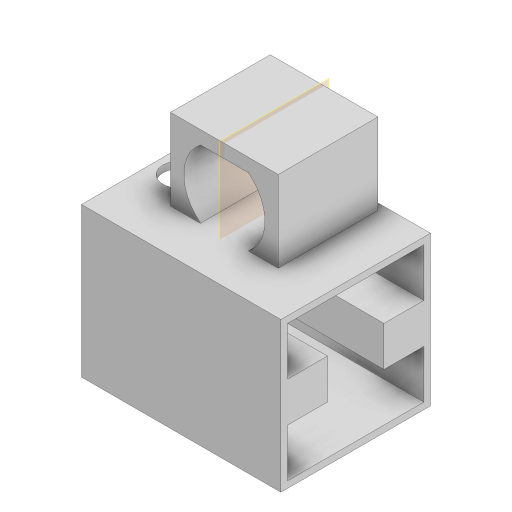
# Autodesk Inventor part: motor mount left
Saved by Autodesk Inventor 2023 (Build 270158000, 158)
## iProperties
Created: 2023-07-19
Part Number: motor mount left
Material: Generic
Document SubType Name: Modeling
Designer: Juyoung Han
Density: 1 g/cm^3
Appearance: Default
Author: Juyoung Han
Autodesk Inventor part; units mm, degrees
ref_plane "YZ Plane" through (0, 0, 0) normal (1, 0, 0) x (0, 1, 0)
ref_plane "XZ Plane" through (0, 0, 0) normal (0, 1, 0) x (-1, 0, 0)
ref_plane "XY Plane" through (0, 0, 0) normal (0, 0, 1) x (1, 0, 0)
sketch "Sketch4" plane through (0, 0, 0) normal (0, 0, 1) x (1, 0, 0)
  arc A0 (2.5, 0) -> (2.5, -10.2) centre (6.452, -5.1) ccw
  arc A1 (9.7, -10.2) -> (9.7, 0) centre (5.748, -5.1) ccw
  line L0 (-2, 2) -> (14.2, 2)
  line L1 (14.2, 2) -> (14.2, -10.2)
  line L2 (-2, -10.2) -> (-2, 2)
  line L3 (-2, -10.2) -> (2.5, -10.2)
  line L4 (9.7, -10.2) -> (14.2, -10.2)
  line L5 (2.5, 0) -> (9.7, 0)
  point P0 (0, 0)
  point P1 (6.1, 0)
  point P2 (6.1, -10.2)
  dimension "d50" = 3.6
  dimension "d51" = 3.6
  dimension "d52" = 3.6
  dimension "d53" = 3.6
  constraints: 12 end point, 4 point on circle, 2 centre point, 1 horizontal, 1 parallel, 1 perpendicular, 1 point on line
  measures "d50" distance of L5.start point (6.1, 0)
  measures "d51" distance of point (6.1, 0) L5.end
  measures "d52" distance of point (6.1, -10.2) L3.end
  measures "d53" distance of point (6.1, -10.2) L4.start
extrude "Extrusion4" add sketch "Sketch4" along normal blind 15
ref_plane "Work Plane2" through (6.1, -10.2, 0) normal (1, 0, 0) x (0, 0, -1)
sketch "Sketch5" plane through (6.1, -10.2, 0) normal (1, 0, 0) x (0, 0, -1)
  line L0 (0, 0) -> (0, 12.2) projected
  line L1 (0, 12.2) -> (-15, 12.2) projected
  line L2 (-15, 0) -> (-15, 12.2) projected
  line L3 (0, 0) -> (-15, 0) projected
  line L4 (1, 0) -> (-21.5, 0)
  line L5 (-21.5, 0) -> (-21.5, -22.5)
  line L6 (-21.5, -22.5) -> (1, -22.5)
  line L7 (1, -22.5) -> (1, 0)
  line L8 (-20.5, -1) -> (0, -1)
  line L9 (0, -21.5) -> (-20.5, -21.5)
  line L10 (-20.5, -8.25) -> (-14.5, -8.25)
  line L11 (-14.5, -8.25) -> (-14.5, -14.25)
  line L12 (-14.5, -14.25) -> (-20.5, -14.25)
  line L13 (0, -8.25) -> (-6, -8.25)
  line L14 (-6, -8.25) -> (-6, -14.25)
  line L15 (-6, -14.25) -> (0, -14.25)
  line L16 (-20.5, -21.5) -> (-20.5, -14.25)
  line L17 (-20.5, -8.25) -> (-20.5, -1)
  line L18 (0, -1) -> (0, -8.25)
  line L19 (0, -14.25) -> (0, -21.5)
  point P0 (0, 10.2)
  point P1 (-20.5, -11.25)
  point P2 (-20.5, -11.25)
  dimension "d58" = 22.5
  dimension "d59" = 22.5
  dimension "d60" = 1
  dimension "d61" = 1
  constraints: 32 end point, 9 parallel, 5 perpendicular, 3 horizontal, 1 point on line
  measures "d58" distance of L6.end L5.end
  measures "d59" distance of L5.end L4.end
  measures "d60" distance from line of L0.start L7
  measures "d61" distance between parallel lines of L4 L8
extrude "Extrusion5" add sketch "Sketch5" along normal mid plane 30 contours L4 L7 L6 L5 L3
sketch "Sketch6" plane through (-8.9, -10.2, 21.5) normal (0, 1, 0) x (1, 0, 0)
  circle A0 centre (3.5, 11.25) radius 2.5
  line L0 (0, 0) -> (0, 22.5) projected
  point P0 (8.9, 21.5)
  dimension "d69" = 5
  dimension "d70" = 3.5
  constraints: 1 centre point
  measures "d69" diameter of A0
  measures "d70" distance from line of A0.centre L0
extrude "Extrusion6" cut sketch "Sketch6" along normal through all both and the other way through all
body "Solid2"
